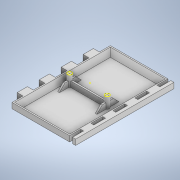
# Autodesk Inventor part: rfid_top
Saved by Autodesk Inventor 2020 (Build 240168000, 168)
## iProperties
Created: 2019-06-30
Part Number: rfid_top
Material: Generic
Document SubType Name: Modeling
Designer: jjsch
Density: 1 g/cm^3
Appearance: Default
Mass: 12.4406 g
Surface Area: 151.295 cm^2
Volume: 12.4406 cm^3
Author: jjsch
Autodesk Inventor part; units mm, degrees
ref_plane "YZ Plane" through (0, 0, 0) normal (1, 0, 0) x (0, 1, 0)
ref_plane "XZ Plane" through (0, 0, 0) normal (0, 1, 0) x (-1, 0, 0)
ref_plane "XY Plane" through (0, 0, 0) normal (0, 0, 1) x (1, 0, 0)
sketch "Sketch1" plane through (0, 0, 0) normal (0, 1, 0) x (-1, 0, 0)
  line L0 (-31.9185, 45) -> (31.9185, 45)
  line L1 (31.9185, 45) -> (31.9185, -45)
  line L2 (31.9185, -45) -> (-31.9185, -45)
  line L3 (-31.9185, -45) -> (-31.9185, 45)
  line L4 (-31.9185, 45) -> (31.9185, -45) construction
  line L5 (31.9185, 45) -> (-31.9185, -45) construction
  point P0 (0, 0)
  dimension "d0" = 63.837
  dimension "d1" = 90
  constraints: 12 end point, 2 midpoint, 2 parallel, 1 horizontal, 1 perpendicular
  measures "d0" distance of L1.end L2.end
  measures "d1" distance of L0.end L1.end
extrude "Extrusion1" add sketch "Sketch1" along normal blind 5
sketch "Sketch2" plane through (0, 5, 0) normal (0, 1, 0) x (1, 0, 0)
  line L0 (31.9185, -45) -> (31.9185, 45) projected
  line L1 (31.9185, -45) -> (26.4995, -45)
  line L2 (26.4995, -45) -> (26.4995, -35)
  line L3 (26.4995, -35) -> (31.9185, -35)
  line L4 (31.9185, -35) -> (31.9185, -45)
  line L5 (-31.9185, 45) -> (-31.9185, -45) projected
  line L6 (-31.9185, -45) -> (-26.4995, -45)
  line L7 (-26.4995, -45) -> (-26.4995, -35)
  line L8 (-26.4995, -35) -> (-31.9185, -35)
  line L9 (-31.9185, -35) -> (-31.9185, -45)
  line L10 (31.9185, -25) -> (26.4995, -25)
  line L11 (26.4995, -25) -> (26.4995, -15)
  line L12 (26.4995, -15) -> (31.9185, -15)
  line L13 (31.9185, -15) -> (31.9185, -25)
  line L14 (-31.9185, -25) -> (-26.4995, -25)
  line L15 (-26.4995, -25) -> (-26.4995, -15)
  line L16 (-26.4995, -15) -> (-31.9185, -15)
  line L17 (-31.9185, -15) -> (-31.9185, -25)
  line L18 (31.9185, -5) -> (26.4995, -5)
  line L19 (26.4995, -5) -> (26.4995, 5)
  line L20 (26.4995, 5) -> (31.9185, 5)
  line L21 (31.9185, 5) -> (31.9185, -5)
  line L22 (-31.9185, -5) -> (-26.4995, -5)
  line L23 (-26.4995, -5) -> (-26.4995, 5)
  line L24 (-26.4995, 5) -> (-31.9185, 5)
  line L25 (-31.9185, 5) -> (-31.9185, -5)
  line L26 (31.9185, 15) -> (26.4995, 15)
  line L27 (26.4995, 15) -> (26.4995, 25)
  line L28 (26.4995, 25) -> (31.9185, 25)
  line L29 (31.9185, 25) -> (31.9185, 15)
  line L30 (-31.9185, 15) -> (-26.4995, 15)
  line L31 (-26.4995, 15) -> (-26.4995, 25)
  line L32 (-26.4995, 25) -> (-31.9185, 25)
  line L33 (-31.9185, 25) -> (-31.9185, 15)
  line L34 (31.9185, 35) -> (26.4995, 35)
  line L35 (26.4995, 35) -> (26.4995, 45)
  line L36 (26.4995, 45) -> (31.9185, 45)
  line L37 (31.9185, 45) -> (31.9185, 35)
  line L38 (-31.9185, 35) -> (-26.4995, 35)
  line L39 (-26.4995, 35) -> (-26.4995, 45)
  line L40 (-26.4995, 45) -> (-31.9185, 45)
  line L41 (-31.9185, 45) -> (-31.9185, 35)
  point P0 (0, 0)
  dimension "d4" = 5.419
  dimension "d5" = 10
  dimension "d6" = 5.419
  dimension "d7" = 10
  dimension "d10" = 20
  constraints: 80 end point, 4 parallel, 2 horizontal, 2 perpendicular, 1 vertical, 64 other
  measures "d4" distance of L2.end L3.end
  measures "d5" distance of L1.end L2.end
  measures "d6" distance of L8.end L7.end
  measures "d7" distance of L7.end L6.end
  measures "d10" distance of L2.end L11.end
extrude "Extrusion2" cut sketch "Sketch2" against normal blind 5
sketch "Sketch3" plane through (0, 5, 0) normal (0, 1, 0) x (1, 0, 0)
  line L0 (28.4995, -45) -> (31.9185, -45)
  line L1 (31.9185, -45) -> (31.9185, 45)
  line L2 (31.9185, 45) -> (28.4995, 45)
  line L3 (28.4995, 45) -> (28.4995, -45)
  line L4 (-26.4995, -45) -> (26.4995, -45) projected
  line L5 (26.4995, -45) -> (26.4995, -35) projected
  point P0 (0, 0)
  dimension "d17" = 90
  dimension "d18" = 3.419
  dimension "d19" = 0
  dimension "d20" = 2
  constraints: 8 end point, 2 parallel, 1 horizontal, 1 perpendicular
  measures "d17" distance of L1.end L0.end
  measures "d18" distance of L0.start L0.end
  measures "d19" distance between parallel lines of L4 L0
  measures "d20" distance between parallel lines of L5 L3
extrude "Extrusion3" add sketch "Sketch3" against normal blind 5
sketch "Sketch4" plane through (0, 5, 0) normal (0, 1, 0) x (1, 0, 0)
  line L0 (31.9185, -45) -> (31.9185, 45) projected
  line L1 (31.9185, 45) -> (28.4995, 45) projected
  line L2 (28.4995, 45) -> (28.4995, 35) projected
  line L3 (28.4995, 35) -> (26.4995, 35) projected
  line L4 (26.4995, 35) -> (26.4995, 45) projected
  line L5 (26.4995, 45) -> (-26.4995, 45) projected
  line L6 (-26.4995, 45) -> (-26.4995, 35) projected
  line L7 (-26.4995, 35) -> (-31.9185, 35) projected
  line L8 (-31.9185, 35) -> (-31.9185, 25) projected
  line L9 (-31.9185, 25) -> (-26.4995, 25) projected
  line L10 (-26.4995, 25) -> (-26.4995, 15) projected
  line L11 (-26.4995, 15) -> (-31.9185, 15) projected
  line L12 (-31.9185, 15) -> (-31.9185, 5) projected
  line L13 (-31.9185, 5) -> (-26.4995, 5) projected
  line L14 (-26.4995, 5) -> (-26.4995, -5) projected
  line L15 (-26.4995, -5) -> (-31.9185, -5) projected
  line L16 (-31.9185, -5) -> (-31.9185, -15) projected
  line L17 (-31.9185, -15) -> (-26.4995, -15) projected
  line L18 (-26.4995, -15) -> (-26.4995, -25) projected
  line L19 (-26.4995, -25) -> (-31.9185, -25) projected
  line L20 (-31.9185, -25) -> (-31.9185, -35) projected
  line L21 (-31.9185, -35) -> (-26.4995, -35) projected
  line L22 (-26.4995, -35) -> (-26.4995, -45) projected
  line L23 (-26.4995, -45) -> (26.4995, -45) projected
  line L24 (26.4995, -45) -> (26.4995, -35) projected
  line L25 (26.4995, -35) -> (28.4995, -35) projected
  line L26 (28.4995, -35) -> (28.4995, -45) projected
  line L27 (28.4995, -45) -> (31.9185, -45) projected
  line L28 (28.4995, 25) -> (28.4995, 15) projected
  line L29 (28.4995, 15) -> (26.4995, 15) projected
  line L30 (26.4995, 15) -> (26.4995, 25) projected
  line L31 (26.4995, 25) -> (28.4995, 25) projected
  line L32 (28.4995, 5) -> (28.4995, -5) projected
  line L33 (28.4995, -5) -> (26.4995, -5) projected
  line L34 (26.4995, -5) -> (26.4995, 5) projected
  line L35 (26.4995, 5) -> (28.4995, 5) projected
  line L36 (28.4995, -15) -> (28.4995, -25) projected
  line L37 (28.4995, -25) -> (26.4995, -25) projected
  line L38 (26.4995, -25) -> (26.4995, -15) projected
  line L39 (26.4995, -15) -> (28.4995, -15) projected
  line L40 (-20.9995, 39.5) -> (20.9995, 39.5)
  line L41 (20.9995, 39.5) -> (20.9995, 29.5)
  line L42 (20.9995, 29.5) -> (26.4185, 29.5)
  line L43 (26.4185, 29.5) -> (26.4185, -29.5)
  line L44 (26.4185, -29.5) -> (20.9995, -29.5)
  line L45 (20.9995, -29.5) -> (20.9995, -39.5)
  line L46 (20.9995, -39.5) -> (-20.9995, -39.5)
  line L47 (-20.9995, -39.5) -> (-20.9995, -30.5)
  line L48 (-20.9995, -30.5) -> (-20.9995, -10.5)
  line L49 (-20.9995, -10.5) -> (-20.9995, 9.5)
  line L50 (-20.9995, 9.5) -> (-20.9995, 29.5)
  line L51 (-20.9995, 29.5) -> (-20.9995, 39.5)
  line L52 (20.9995, 29.5) -> (20.9995, -29.5)
  point P0 (0, 0)
  dimension "d23" = 5.5
  constraints: 26 end point, 1 collinear, 11 other
  measures "d23" distance between parallel lines of L5 L40
extrude "Extrusion4" cut sketch "Sketch4" against normal blind 4 contours L40 L41 L52 L45 L46 L47 L48 L49 L50 L51
chamfer "Chamfer1" distance 4 angle 45 4 edges at (-20.9995, 5, 0) (0, 5, -39.5) (20.9995, 5, 0) (0, 5, 39.5)
sketch "Sketch5" plane through (0, 0, 0) normal (0, -1, 0) x (1, 0, 0)
  circle A0 centre (-17.05, 1.5) radius 1.9
  circle A1 centre (17.05, 1.5) radius 1.9
  line L0 (-26.4995, 45) -> (26.4995, 45) projected
  line L1 (26.4995, -45) -> (-26.4995, -45) projected
  point P0 (0, 0)
  dimension "d33" = 3.8
  dimension "d34" = 3.8
  dimension "d61" = 17.05
  dimension "d62" = 17.05
  dimension "d63" = 1.5
  constraints: 2 centre point, 1 horizontal alignment
  measures "d33" diameter of A0
  measures "d34" diameter of A1
  measures "d61" horizontal distance of point (0, 0) A0.centre
  measures "d62" horizontal distance of point (0, 0) A1.centre
  measures "d63" vertical distance of point (0, 0) A0.centre
extrude "Extrusion5" add sketch "Sketch5" against normal blind 15
sketch "Sketch7" plane through (17.05, 15, 1.5) normal (0, 1, 0) x (1, 0, 0)
  circle A0 centre (-34.1, 0) radius 1.9 projected
  circle A1 centre (0, 0) radius 1.9 projected
  point P0 (-17.05, 1.5)
extrude "Extrusion7" cut sketch "Sketch7" against normal blind 4
sketch "Sketch8" plane through (-17.05, 11, 1.5) normal (0, 1, 0) x (1, 0, 0)
  circle A0 centre (34.1, 0) radius 1.9 projected
  circle A1 centre (0, 0) radius 1.9 projected
  point P0 (17.05, 1.5)
  constraints: 2 coincident
sketch "Sketch9" plane through (0, 5, 0) normal (0, 1, 0) x (1, 0, 0)
  line L0 (28.4995, -15) -> (28.4995, -25) projected
  line L1 (28.4995, -25) -> (26.4995, -25) projected
  line L2 (26.4995, -25) -> (26.4995, -15) projected
  line L3 (26.4995, -15) -> (28.4995, -15) projected
  line L4 (28.4995, 5) -> (28.4995, -5) projected
  line L5 (28.4995, -5) -> (26.4995, -5) projected
  line L6 (26.4995, -5) -> (26.4995, 5) projected
  line L7 (26.4995, 5) -> (28.4995, 5) projected
  line L8 (28.4995, 25) -> (28.4995, 15) projected
  line L9 (28.4995, 15) -> (26.4995, 15) projected
  line L10 (26.4995, 15) -> (26.4995, 25) projected
  line L11 (26.4995, 25) -> (28.4995, 25) projected
  line L12 (31.9185, -45) -> (31.9185, 45) projected
  line L13 (31.9185, 45) -> (28.4995, 45) projected
  line L14 (28.4995, 45) -> (28.4995, 35) projected
  line L15 (28.4995, 35) -> (26.4995, 35) projected
  line L16 (26.4995, 35) -> (26.4995, 45) projected
  line L17 (26.4995, 45) -> (-26.4995, 45) projected
  line L18 (-26.4995, 45) -> (-26.4995, 35) projected
  line L19 (-26.4995, 35) -> (-31.9185, 35) projected
  line L20 (-31.9185, 35) -> (-31.9185, 25) projected
  line L21 (-31.9185, 25) -> (-26.4995, 25) projected
  line L22 (-26.4995, 25) -> (-26.4995, 15) projected
  line L23 (-26.4995, 15) -> (-31.9185, 15) projected
  line L24 (-31.9185, 15) -> (-31.9185, 5) projected
  line L25 (-31.9185, 5) -> (-26.4995, 5) projected
  line L26 (-26.4995, 5) -> (-26.4995, -5) projected
  line L27 (-26.4995, -5) -> (-31.9185, -5) projected
  line L28 (-31.9185, -5) -> (-31.9185, -15) projected
  line L29 (-31.9185, -15) -> (-26.4995, -15) projected
  line L30 (-26.4995, -15) -> (-26.4995, -25) projected
  line L31 (-26.4995, -25) -> (-31.9185, -25) projected
  line L32 (-31.9185, -25) -> (-31.9185, -35) projected
  line L33 (-31.9185, -35) -> (-26.4995, -35) projected
  line L34 (-26.4995, -35) -> (-26.4995, -45) projected
  line L35 (-26.4995, -45) -> (26.4995, -45) projected
  line L36 (26.4995, -45) -> (26.4995, -35) projected
  line L37 (26.4995, -35) -> (28.4995, -35) projected
  line L38 (28.4995, -35) -> (28.4995, -45) projected
  line L39 (28.4995, -45) -> (31.9185, -45) projected
  line L40 (24.9995, 43.5) -> (-24.9995, 43.5) projected
  line L41 (24.9995, -43.5) -> (24.9995, 43.5) projected
  line L42 (-24.9995, -43.5) -> (24.9995, -43.5) projected
  line L43 (-24.9995, 43.5) -> (-24.9995, -43.5) projected
  line L44 (31.6185, 44.7) -> (31.6185, -44.7)
  line L45 (31.6185, -44.7) -> (28.7995, -44.7)
  line L46 (28.7995, -44.7) -> (28.7995, -34.7)
  line L47 (28.7995, -34.7) -> (26.1995, -34.7)
  line L48 (26.1995, -34.7) -> (26.1995, -44.7)
  line L49 (26.1995, -44.7) -> (-26.1995, -44.7)
  line L50 (-26.1995, -44.7) -> (-26.1995, -34.7)
  line L51 (-26.1995, -34.7) -> (-31.6185, -34.7)
  line L52 (-31.6185, -34.7) -> (-31.6185, -25.3)
  line L53 (-31.6185, -25.3) -> (-26.1995, -25.3)
  line L54 (-26.1995, -25.3) -> (-26.1995, -14.7)
  line L55 (-26.1995, -14.7) -> (-31.6185, -14.7)
  line L56 (-31.6185, -14.7) -> (-31.6185, -5.3)
  line L57 (-31.6185, -5.3) -> (-26.1995, -5.3)
  line L58 (-26.1995, -5.3) -> (-26.1995, 5.3)
  line L59 (-26.1995, 5.3) -> (-31.6185, 5.3)
  line L60 (-31.6185, 5.3) -> (-31.6185, 14.7)
  line L61 (-31.6185, 14.7) -> (-26.1995, 14.7)
  line L62 (-26.1995, 14.7) -> (-26.1995, 25.3)
  line L63 (-26.1995, 25.3) -> (-31.6185, 25.3)
  line L64 (-31.6185, 25.3) -> (-31.6185, 34.7)
  line L65 (-31.6185, 34.7) -> (-26.1995, 34.7)
  line L66 (-26.1995, 34.7) -> (-26.1995, 44.7)
  line L67 (-26.1995, 44.7) -> (26.1995, 44.7)
  line L68 (26.1995, 44.7) -> (26.1995, 34.7)
  line L69 (26.1995, 34.7) -> (28.7995, 34.7)
  line L70 (28.7995, 34.7) -> (28.7995, 44.7)
  line L71 (28.7995, 44.7) -> (31.6185, 44.7)
  line L72 (28.7995, -25.3) -> (28.7995, -14.7)
  line L73 (28.7995, -14.7) -> (26.1995, -14.7)
  line L74 (26.1995, -14.7) -> (26.1995, -25.3)
  line L75 (26.1995, -25.3) -> (28.7995, -25.3)
  line L76 (28.7995, -5.3) -> (28.7995, 5.3)
  line L77 (28.7995, 5.3) -> (26.1995, 5.3)
  line L78 (26.1995, 5.3) -> (26.1995, -5.3)
  line L79 (26.1995, -5.3) -> (28.7995, -5.3)
  line L80 (26.1995, 25.3) -> (26.1995, 14.7)
  line L81 (26.1995, 14.7) -> (28.7995, 14.7)
  line L82 (28.7995, 14.7) -> (28.7995, 25.3)
  line L83 (28.7995, 25.3) -> (26.1995, 25.3)
  line L84 (28.4995, -15) -> (28.4995, -25) projected
  line L85 (28.4995, -25) -> (26.4995, -25) projected
  line L86 (26.4995, -25) -> (26.4995, -15) projected
  line L87 (26.4995, -15) -> (28.4995, -15) projected
  line L88 (28.4995, 5) -> (28.4995, -5) projected
  line L89 (28.4995, -5) -> (26.4995, -5) projected
  line L90 (26.4995, -5) -> (26.4995, 5) projected
  line L91 (26.4995, 5) -> (28.4995, 5) projected
  line L92 (28.4995, 25) -> (28.4995, 15) projected
  line L93 (28.4995, 15) -> (26.4995, 15) projected
  line L94 (26.4995, 15) -> (26.4995, 25) projected
  line L95 (26.4995, 25) -> (28.4995, 25) projected
  line L96 (31.9185, -45) -> (31.9185, 45) projected
  line L97 (31.9185, 45) -> (28.4995, 45) projected
  line L98 (28.4995, 45) -> (28.4995, 35) projected
  line L99 (28.4995, 35) -> (26.4995, 35) projected
  line L100 (26.4995, 35) -> (26.4995, 45) projected
  line L101 (26.4995, 45) -> (-26.4995, 45) projected
  line L102 (-26.4995, 45) -> (-26.4995, 35) projected
  line L103 (-26.4995, 35) -> (-31.9185, 35) projected
  line L104 (-31.9185, 35) -> (-31.9185, 25) projected
  line L105 (-31.9185, 25) -> (-26.4995, 25) projected
  line L106 (-26.4995, 25) -> (-26.4995, 15) projected
  line L107 (-26.4995, 15) -> (-31.9185, 15) projected
  line L108 (-31.9185, 15) -> (-31.9185, 5) projected
  line L109 (-31.9185, 5) -> (-26.4995, 5) projected
  line L110 (-26.4995, 5) -> (-26.4995, -5) projected
  line L111 (-26.4995, -5) -> (-31.9185, -5) projected
  line L112 (-31.9185, -5) -> (-31.9185, -15) projected
  line L113 (-31.9185, -15) -> (-26.4995, -15) projected
  line L114 (-26.4995, -15) -> (-26.4995, -25) projected
  line L115 (-26.4995, -25) -> (-31.9185, -25) projected
  line L116 (-31.9185, -25) -> (-31.9185, -35) projected
  line L117 (-31.9185, -35) -> (-26.4995, -35) projected
  line L118 (-26.4995, -35) -> (-26.4995, -45) projected
  line L119 (-26.4995, -45) -> (26.4995, -45) projected
  line L120 (26.4995, -45) -> (26.4995, -35) projected
  line L121 (26.4995, -35) -> (28.4995, -35) projected
  line L122 (28.4995, -35) -> (28.4995, -45) projected
  line L123 (28.4995, -45) -> (31.9185, -45) projected
  line L124 (24.9995, 43.5) -> (-24.9995, 43.5) projected
  line L125 (24.9995, -43.5) -> (24.9995, 43.5) projected
  line L126 (-24.9995, -43.5) -> (24.9995, -43.5) projected
  line L127 (-24.9995, 43.5) -> (-24.9995, -43.5) projected
  point P0 (0, 0)
  dimension "d55" = 0.3
  dimension "d56" = 0.3
  dimension "d57" = 0.3
  dimension "d58" = 0.3
  constraints: 80 end point, 36 other
  measures "d55" distance between parallel lines of L12 L44
  measures "d56" distance between parallel lines of L0 L72
  measures "d57" distance between parallel lines of L4 L76
  measures "d58" distance between parallel lines of L10 L80
extrude "Tolerances Extrusion" cut sketch "Sketch9" against normal blind 5 contours L0 L1 L2 L3 | L4 L5 L6 L7 | L8 L9 L10 L11 | L39 L38 L37 L36 L35 L34 L33 L32 L31 L30 L29 L28 L27 L26 L25 L24 L23 L22 L21 L20 L19 L18 L17 L16 L15 L14 L13 L12 | L75 L74 L73 L72 | L79 L78 L77 L76 | L83 L82 L81 L80
sketch "Sketch10" plane through (0, 1, 0) normal (0, 1, 0) x (1, 0, 0)
  line L0 (17.05, -0.772) -> (-17.05, -0.772)
  line L1 (-17.05, -0.772) -> (-17.05, -2.228)
  line L2 (-17.05, -2.228) -> (17.05, -2.228)
  line L3 (17.05, -2.228) -> (17.05, -0.772)
  line L4 (17.05, -0.772) -> (-17.05, -2.228) construction
  line L5 (-17.05, -0.772) -> (17.05, -2.228) construction
  line L6 (-16.3, -11.5) -> (-17.8, -11.5)
  line L7 (-17.8, -11.5) -> (-17.8, 8.5)
  line L8 (-17.8, 8.5) -> (-16.3, 8.5)
  line L9 (-16.3, 8.5) -> (-16.3, -11.5)
  line L10 (-16.3, -11.5) -> (-17.8, 8.5) construction
  line L11 (-17.8, -11.5) -> (-16.3, 8.5) construction
  line L12 (17.8, -11.5) -> (16.3, -11.5)
  line L13 (16.3, -11.5) -> (16.3, 8.5)
  line L14 (16.3, 8.5) -> (17.8, 8.5)
  line L15 (17.8, 8.5) -> (17.8, -11.5)
  line L16 (17.8, -11.5) -> (16.3, 8.5) construction
  line L17 (16.3, -11.5) -> (17.8, 8.5) construction
  point P0 (0, 0)
  point P1 (0, -1.5)
  point P2 (-17.05, -1.5)
  point P3 (17.05, -1.5)
  point P4 (16.3, -0.772)
  point P5 (16.3, -2.228)
  point P6 (-16.3, -2.228)
  point P7 (-16.3, -0.772)
  dimension "d66" = 1.5
  dimension "d67" = 20
  dimension "d68" = 1.5
  dimension "d69" = 20
  constraints: 36 end point, 8 midpoint, 6 parallel, 3 horizontal, 3 perpendicular
  measures "d66" distance of L7.end L8.end
  measures "d67" distance of L6.end L7.end
  measures "d68" distance of L13.end L14.end
  measures "d69" distance of L12.end L13.end
extrude "Extrusion9" add sketch "Sketch10" along normal blind 5
chamfer "Chamfer2" distance 5 angle 45 5 edges at (-17.05, 6, 11.5) (17.05, 6, 11.5) (17.05, 6, -8.5) (-16.3, 3.5, -8.5) (-17.05, 6, -8.5)
body "Solid1"
